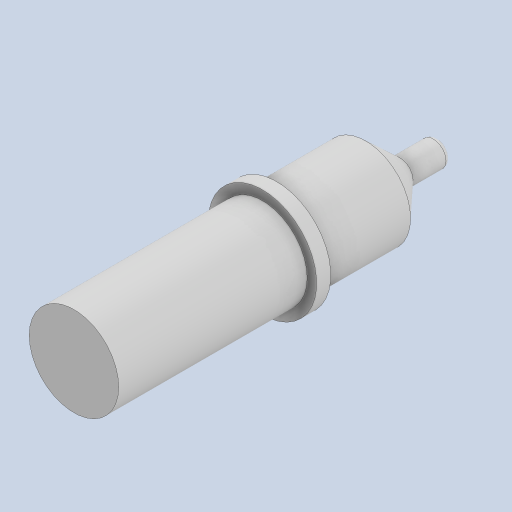
# Autodesk Inventor part: Marcador_V2
Saved by Autodesk Inventor 2024 (Build 280153000, 153)
## iProperties
Created: 2025-06-11
Part Number: Marcador_V2
Material: Genérico
Document SubType Name: Modeling
Designer: ANDRES
Density: 1 g/cm^3
Appearance: Valor por defecto
Author: ANDRES
Autodesk Inventor part; units mm, degrees
ref_plane "YZ Plane" through (0, 0, 0) normal (1, 0, 0) x (0, 1, 0)
ref_plane "XZ Plane" through (0, 0, 0) normal (0, 1, 0) x (-1, 0, 0)
ref_plane "XY Plane" through (0, 0, 0) normal (0, 0, 1) x (1, 0, 0)
sketch "Boceto1" plane through (0, 0, 0) normal (0, 1, 0) x (-1, 0, 0)
  line L0 (9.5, -37.26) -> (9.5, 0)
  line L1 (0, 20.9781) -> (0, -29.6058) construction
  line L2 (0, -29.26) -> (2.7, -29.26)
  line L3 (2.7, -29.26) -> (2.7, -37.26)
  line L4 (2.7, -37.26) -> (0, -37.26)
  line L5 (0, -37.26) -> (0, -29.26)
  line L6 (2.7, -29.26) -> (9.5, -21.9279)
  line L7 (9.5, 0) -> (11.5, 0)
  line L8 (11.5, 0) -> (11.5, -3)
  line L9 (11.5, -3) -> (9.5, -3)
  line L10 (9.5, -3) -> (9.5, 0)
  line L11 (9.5, 0) -> (0, 0)
  line L12 (0, 0) -> (0, 40)
  line L13 (0, 40) -> (9.5, 40)
  line L14 (9.5, 40) -> (9.5, 0)
  line L15 (0, 40) -> (0, -37.26)
  dimension "d0" = 9.5
  dimension "d1" = 37.26
  dimension "d2" = 2.7
  dimension "d3" = 8
  dimension "d4" = 10
  dimension "d5" = 2
  dimension "d6" = 3
  dimension "d7" = 40
  constraints: 32 end point, 6 parallel, 4 vertical, 3 horizontal, 3 perpendicular, 3 point on line, 2 horizontal alignment
  measures "d0" distance between parallel lines of L1 L0
  measures "d1" distance of L0.start L0.end
  measures "d2" distance of L3.end L4.end
  measures "d3" distance of L2.end L3.end
  measures "d4" distance of L2.end L6.end
  measures "d5" distance of L8.end L9.end
  measures "d6" distance of L7.end L8.end
  measures "d7" distance of L11.end L12.end
revolve "Revolución1" add sketch "Boceto1" angle 360 about axis through (0, 0, 40) along (0, 0, -1)
fillet "Empalme1" radius 1 1 edges at (2.7, 0, -37.26)
